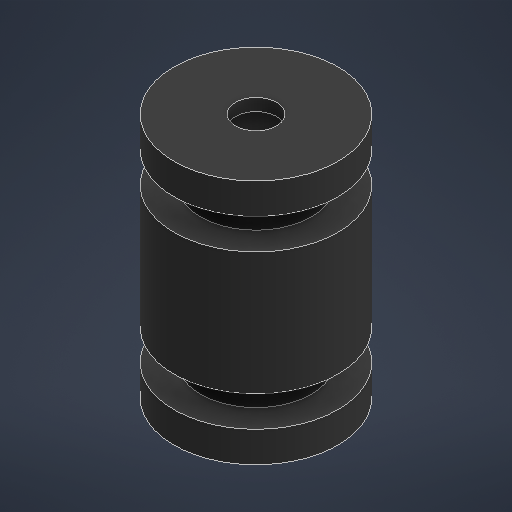
# Autodesk Inventor part: antivibracion
Saved by Autodesk Inventor 2026 (Build 300175050, 175E)
## iProperties
Created: 2025-06-30
Part Number: antivibracion
Material: Caucho
Document SubType Name: Modeling
Designer: rodri
Density: 0.93 g/cm^3
Appearance: Caucho - Negro
Author: rodri
## iProperties of the stored document antivibracion_3DPrint.ipt
Created: 2025-06-30
Part Number: antivibracion_3DPrint
Material: Genérico
Document SubType Name: Modeling
Designer: rodri
Density: 1 g/cm^3
Appearance: Valor por defecto
Author: rodri
Autodesk Inventor part; units mm, degrees
ref_plane "YZ Plane" through (0, 0, 0) normal (1, 0, 0) x (0, 1, 0)
ref_plane "XZ Plane" through (0, 0, 0) normal (0, 1, 0) x (-1, 0, 0)
sketch "Boceto1" plane through (0, 0, 0) normal (0, 1, 0) x (-1, 0, 0)
  circle A0 centre (0, 0) radius 4
  circle A1 centre (0, 0) radius 1
  dimension "d0" = 8
  dimension "d7" = 2
  constraints: 2 centre point, 2 coincident
  measures "d0" diameter of A0
  measures "d7" diameter of A1
extrude "Extrusión1" add sketch "Boceto1" along normal mid plane 12 contours A0 | A1
ref_plane "Plano de trabajo1" through (0, 4.5, 0) normal (0, 1, 0) x (1, 0, 0)
sketch "Boceto2" plane through (0, 4.5, 0) normal (0, 1, 0) x (1, 0, 0)
  circle A0 centre (0, 0) radius 4 projected
  circle A1 centre (0, 0) radius 2.7
  dimension "d4" = 5.4
  constraints: 1 centre point, 1 coincident
  measures "d4" diameter of A1
extrude "Extrusión2" cut sketch "Boceto2" against normal blind 1.5
mirror "Simetría1" about plane through (0, 0, 0) normal (0, 1, 0) of "Extrusión2"
shell "Vaciado2" thickness 0.6 removed faces 0
sketch "Boceto4" plane through (0, 6, 0) normal (0, 1, 0) x (1, 0, 0)
  circle A0 centre (0, 0) radius 1
  dimension "d14" = 2
  constraints: 1 centre point, 1 coincident
  measures "d14" diameter of A0
extrude "Extrusión4" cut sketch "Boceto4" against normal through all
